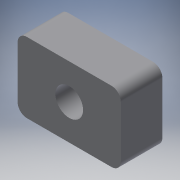
# Autodesk Inventor part: ConnectingBlockTail
Saved by Autodesk Inventor 2016 (Build 200138000, 138)
## iProperties
Created: 2017-03-10
Part Number: ConnectingBlockTail
Material: Generic
Document SubType Name: Modeling
Designer: Owner
Density: 1 g/cm^3
Appearance: Default
Author: Owner
Autodesk Inventor part; units mm, degrees
ref_plane "YZ Plane" through (0, 0, 0) normal (1, 0, 0) x (0, 1, 0)
ref_plane "XZ Plane" through (0, 0, 0) normal (0, 1, 0) x (-1, 0, 0)
ref_plane "XY Plane" through (0, 0, 0) normal (0, 0, 1) x (1, 0, 0)
sketch "Sketch1" plane through (0, 0, 0) normal (0, 0, 1) x (1, 0, 0)
  circle A0 centre (14.22, 3.81) radius 1.5 projected
  circle A1 centre (14.22, -4.69) radius 1.5 projected
  line L0 (8.6298, -8.5) -> (19.8102, -8.5) projected
  line L1 (19.8102, -8.5) -> (19.8102, 0) projected
  line L2 (19.8102, 0) -> (8.6298, 0) projected
  line L3 (8.6298, 0) -> (8.6298, -8.5) projected
  line L4 (8.6298, 0) -> (19.8102, 0)
  line L5 (19.8102, 0) -> (19.8102, 7.62)
  line L6 (19.8102, 7.62) -> (8.6298, 7.62)
  line L7 (8.6298, 7.62) -> (8.6298, 0)
  point P0 (0, 0)
  dimension "d0" = 3.81
  constraints: 8 end point, 2 parallel, 1 horizontal, 1 perpendicular
  measures "d0" distance from line of L6 A0.centre
extrude "Extrusion1" add sketch "Sketch1" along normal blind 4.5 contours L7 L6 L5 L2
fillet "Fillet1" radius 1 4 edges at (8.6298, 7.62, 2.25) (8.6298, 0, 2.25) (19.8102, 7.62, 2.25) (19.8102, 0, 2.25)
body "Solid1"
